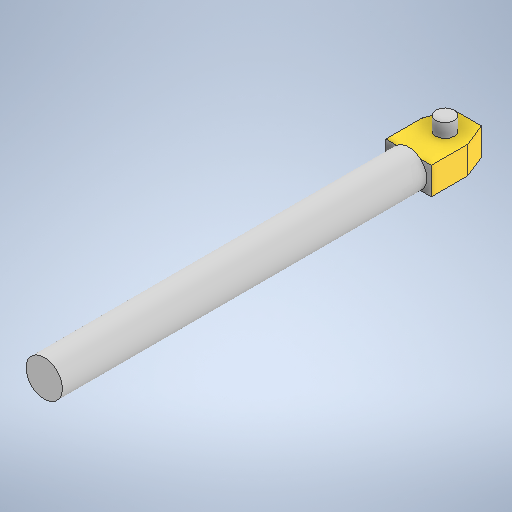
# Autodesk Inventor part: Parth_Pushrod
Saved by Autodesk Inventor 2025 (Build 290162000, 162)
## iProperties
Created: 2024-11-03
Part Number: Parth_Pushrod
Material: Generic
Document SubType Name: Modeling
Designer: kalep
Density: 1 g/cm^3
Appearance: Default
Author: kalep
Autodesk Inventor part; units mm, degrees
ref_plane "YZ Plane" through (0, 0, 0) normal (1, 0, 0) x (0, 1, 0)
ref_plane "XZ Plane" through (0, 0, 0) normal (0, 1, 0) x (-1, 0, 0)
ref_plane "XY Plane" through (0, 0, 0) normal (0, 0, 1) x (1, 0, 0)
sketch "Sketch1" plane through (0, 0, 0) normal (0, 0, 1) x (1, 0, 0)
  circle A0 centre (0, 0) radius 20
  dimension "d0" = 40
  constraints: 1 centre point, 1 coincident
  measures "d0" diameter of A0
extrude "Extrusion1" add sketch "Sketch1" along normal blind 400
sketch "Sketch2" plane through (0, 0, 0) normal (0, 1, 0) x (-1, 0, 0)
  line L0 (15, -65) -> (-15, -65)
  line L1 (-25, -40) -> (-25, 0)
  line L2 (-25, 0) -> (25, 0)
  line L3 (25, 0) -> (25, -40)
  line L4 (25, -65) -> (-25, 0) construction
  line L5 (-25, -65) -> (25, 0) construction
  line L6 (25, -40) -> (15, -65)
  line L7 (-25, -40) -> (-15, -65)
  point P0 (0, 0)
  point P1 (0, -32.5)
  dimension "d3" = 50
  dimension "d4" = 65
  dimension "d5" = 25
  dimension "d6" = 10
  dimension "d7" = 25
  dimension "d8" = 10
  constraints: 16 end point, 4 point on line, 2 midpoint, 2 parallel, 1 horizontal, 1 perpendicular
  measures "d3" distance of L1.end L2.end
  measures "d4" distance of L5.start L1.end
  measures "d5" distance of L3.end L4.start
  measures "d6" distance of L0.start L4.start
  measures "d7" distance of L1.start L5.start
  measures "d8" distance of L0.end L5.start
extrude "Extrusion2" add sketch "Sketch2" along normal mid plane 30
sketch "Sketch3" plane through (0, 15, 0) normal (0, 1, 0) x (1, 0, 0)
  point P0 (0, 0)
sketch "Sketch4" plane through (0, 0, 0) normal (0, 1, 0) x (-1, 0, 0)
  circle A0 centre (0, -40) radius 10
  line L0 (13.2288, 0) -> (-13.2288, 0) projected
  point P0 (0, 0)
  dimension "d11" = 20
  dimension "d12" = 40
  constraints: 1 centre point
  measures "d11" diameter of A0
  measures "d12" distance from line of L0 A0.centre
extrude "Extrusion3" add sketch "Sketch4" along normal mid plane 60
body "Solid1"
